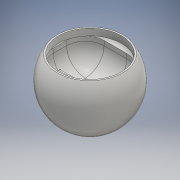
# Autodesk Inventor part: eye ball
Saved by Autodesk Inventor 2016 (Build 200138000, 138)
## iProperties
Created: 2016-03-20
Part Number: eye ball
Material: ABS Plastic
Document SubType Name: Modeling
Designer: Hamid Osooli
Density: 1.06 g/cm^3
Appearance: Smooth - White
Mass: 70.5976 g
Surface Area: 145.278 cm^2
Volume: 66.6016 cm^3
Author: Hamid Osooli
Autodesk Inventor part; units mm, degrees
ref_plane "YZ Plane" through (0, 0, 0) normal (1, 0, 0) x (0, 1, 0)
ref_plane "XZ Plane" through (0, 0, 0) normal (0, 1, 0) x (-1, 0, 0)
ref_plane "XY Plane" through (0, 0, 0) normal (0, 0, 1) x (1, 0, 0)
sketch "Sketch5" plane through (0, 0, 0) normal (1, 0, 0) x (0, 1, 0)
  arc A0 (0, -30) -> (24.5746, 17.2073) centre (0, 0) ccw
  line L0 (0, 0) -> (30, 0) construction
  line L1 (24.5746, 17.2073) -> (0, 17.2073)
  line L2 (0, -30) -> (0, 17.2073)
  point P0 (0, 0)
  dimension "d32" = 30
  constraints: 6 end point, 2 point on circle, 1 centre point, 1 horizontal, 1 vertical
  measures "d32" radius of A0
revolve "Revolution3" add sketch "Sketch5" angle 360 about axis through (0, 0, -30) along (0, 0, 1)
sketch "Sketch7" plane through (0, 0, 17.2073) normal (0, 0, 1) x (1, 0, 0)
  circle A0 centre (0, 0) radius 23.5
  dimension "d40" = 47
  constraints: 1 centre point, 1 coincident
  measures "d40" diameter of A0
extrude "Extrusion4" cut sketch "Sketch7" against normal blind 5
sketch "Sketch10" plane through (0, 0, 12.2073) normal (0, 0, 1) x (1, 0, 0)
  line L0 (-8.5, 19) -> (8.5, 19)
  line L1 (22.5, 5) -> (22.5, -5)
  line L2 (8.5, -19) -> (-8.5, -19)
  line L3 (-22.5, -5) -> (-22.5, 5)
  arc A0 (-8.5, 19) -> (-22.5, 5) centre (-8.5, 5) ccw
  arc A1 (22.5, 5) -> (8.5, 19) centre (8.5, 5) ccw
  arc A2 (8.5, -19) -> (22.5, -5) centre (8.5, -5) ccw
  arc A3 (-22.5, -5) -> (-8.5, -19) centre (-8.5, -5) ccw
  point P0 (0, 0)
  point P1 (-22.5, 19)
  point P2 (22.5, 19)
  point P3 (22.5, -19)
  point P4 (-22.5, -19)
  dimension "d43" = 45
  dimension "d44" = 38
  dimension "d45" = 90
  dimension "d46" = 45
  dimension "d47" = 14
  constraints: 8 end point, 8 point on circle, 8 point on line, 8 tangent, 4 centre point, 3 equal radius, 2 perpendicular, 1 horizontal
  measures "d43" distance of point (-22.5, 19) point (22.5, 19)
  measures "d44" distance of point (22.5, 19) point (22.5, -19)
  measures "d45" angle of L0 L1
  measures "d46" distance of point (22.5, -19) point (-22.5, -19)
  measures "d47" radius of A0
extrude "Extrusion5" cut sketch "Sketch10" against normal blind 17.5
sketch "Sketch11" plane through (0, 0, -5.2927) normal (0, 0, 1) x (1, 0, 0)
  line L0 (-8, -4.5) -> (8, -4.5)
  line L1 (8, -4.5) -> (8, 4.5)
  line L2 (8, 4.5) -> (-8, 4.5)
  line L3 (-8, 4.5) -> (-8, -4.5)
  dimension "d73" = 16
  dimension "d74" = 9
  constraints: 8 end point, 2 parallel, 1 horizontal, 1 perpendicular
  measures "d73" distance of L2.end L1.end
  measures "d74" distance of L1.end L0.end
extrude "Extrusion6" cut sketch "Sketch11" against normal up to next
sketch "Sketch12" plane through (0, 0, -5.2927) normal (0, 0, 1) x (1, 0, 0)
  line L0 (-12.5, -13) -> (12.5, -13)
  line L1 (12.5, -13) -> (12.5, -10)
  line L2 (12.5, -10) -> (-12.5, -10)
  line L3 (-12.5, -10) -> (-12.5, -13)
  point P0 (0, 0)
  dimension "d54" = 25
  dimension "d55" = 3
  constraints: 8 end point, 3 perpendicular, 1 horizontal
  measures "d54" distance of L0.start L0.end
  measures "d55" distance of L0.end L1.end
extrude "Extrusion7" add sketch "Sketch12" along normal blind 12
fillet "Fillet1" radius 14 8 edges at (18.3995, 14.8995, -5.2927) (22.5, 0, -5.2927) (18.3995, -14.8995, -5.2927) (0, -19, -5.2927) (-18.3995, -14.8995, -5.2927) (-22.5, 0, -5.2927) (-18.3995, 14.8995, -5.2927) (0, 19, -5.2927)
fillet "Fillet2" radius 1 8 edges at (-12.5, -10, 1.4823) (12.5, -10, 1.4823) (12.5, -13, 2.3221) (-12.5, -13, 2.3221) (0, -10, 6.7073) (0, -13, 6.7073) (-12.5, -11.5, 6.7073) (12.5, -11.5, 6.7073)
sketch "Sketch13" plane through (-8.5, -10, -4.3694) normal (0, 1, 0) x (1, 0, 0)
  line L0 (17, 0) -> (0, 0) projected
  point P0 (8.5, -7.9415)
  point P1 (8.5, -7.9415)
  constraints: 1 coincident
hole "Hole1" at (0, -10, 3.5721) direction (0, -1, 0) diameter 2.5 end up to surface
sketch "Sketch14" plane through (0, 0, -5.2927) normal (0, 0, 1) x (1, 0, 0)
  circle A0 centre (0, 0) radius 5
  dimension "d70" = 10
  constraints: 1 centre point, 1 coincident
  measures "d70" diameter of A0
extrude "Extrusion8" cut sketch "Sketch14" against normal blind 5 draft -30
body "Solid3"
